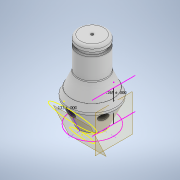
# Autodesk Inventor part: piston badflowchannel-1-16in-thread - neutron - 65flowchan
Saved by Autodesk Inventor 2020 (Build 240168000, 168)
## iProperties
Created: 2022-01-16
Part Number: piston badflowchannel-1-16in-thread - neutron - 65flowchan
Material: Generic
Document SubType Name: Modeling
Designer: pab2
Density: 1 g/cm^3
Appearance: Default
Author: pab2
Autodesk Inventor part; units mm, degrees
ref_plane "YZ Plane" through (0, 0, 0) normal (1, 0, 0) x (0, 1, 0)
ref_plane "XZ Plane" through (0, 0, 0) normal (0, 1, 0) x (-1, 0, 0)
ref_plane "XY Plane" through (0, 0, 0) normal (0, 0, 1) x (1, 0, 0)
sketch "Sketch1" plane through (0, 0, 0) normal (0, 0, 1) x (1, 0, 0)
  line L0 (0, 0) -> (8.4519, 0)
  line L1 (8.4519, 0) -> (8.4519, 12.7)
  line L2 (8.4519, 12.7) -> (7.0041, 12.7)
  line L3 (7.0041, 12.7) -> (7.0041, 15.113)
  line L4 (7.0041, 15.113) -> (8.4519, 15.113)
  line L5 (8.4519, 15.113) -> (8.4519, 18.288)
  line L6 (8.4519, 18.288) -> (0, 18.288)
  line L7 (0, 18.288) -> (0, 0)
  line L8 (0, -36.8534) -> (0, 27.4782) projected
  line L9 (8.4519, 0) -> (8.4519, 6.35)
  line L10 (8.4519, 0) -> (8.4519, 6.35)
  line L11 (8.4519, 6.35) -> (15.4293, -8.6131)
  line L12 (8.4519, 6.35) -> (24.9619, 6.35) construction
  line L13 (15.4293, -8.6131) -> (12.2543, -8.6131)
  line L14 (12.2543, -8.6131) -> (8.4519, 0)
  line L15 (15.4293, -8.6131) -> (0, -8.6131)
  line L16 (0, 0) -> (8.4519, 0)
  line L17 (0, -8.6131) -> (19.05, -8.6131)
  line L18 (19.05, -8.6131) -> (19.05, -27.6631)
  line L19 (19.05, -27.6631) -> (0, -27.6631)
  line L20 (0, -27.6631) -> (0, -8.6131)
  line L21 (19.05, -8.6131) -> (19.05, -16.3778)
  line L22 (7.3425, -27.6631) -> (12.7256, -16.1191)
  line L23 (7.3425, -27.6631) -> (20.0799, -27.6631) construction
  line L24 (8.4519, 0) -> (19.05, -23.5323)
  line L25 (14.2444, -12.862) -> (7.3425, -27.6631)
  point P0 (12.2543, -8.6131)
  point P1 (12.3309, -8.6131)
  dimension "d0" = 8.4519
  dimension "d1" = 12.7
  dimension "d2" = 90
  dimension "d3" = 1.4478
  dimension "d4" = 2.413
  dimension "d5" = 3.175
  dimension "d23" = 16.51
  dimension "d24" = 65
  dimension "d25" = 3.175
  dimension "d83" = 19.05
  dimension "d84" = 19.05
  dimension "d253" = 65
  constraints: 50 end point, 8 perpendicular, 8 point on line, 4 horizontal, 3 parallel, 2 collinear, 2 equal length, 2 vertical, 1 midpoint
  measures "d0" distance of L0.start L0.end
  measures "d1" distance of L0.end L1.end
  measures "d2" angle of L1 L0
  measures "d3" distance of L1.end L2.end
  measures "d4" distance of L2.end L3.end
  measures "d5" distance of L4.end L5.end
  measures "d23" distance of L9.end L11.end
  measures "d24" angle of L11 L12
  measures "d25" distance of L11.end L13.end
  measures "d83" distance of L18.end L19.end
  measures "d84" distance of L17.end L18.end
  measures "d253" angle of L23 L22
revolve "Revolution1" add sketch "Sketch1" angle 360 about axis through (0, -10, 0) along (0, 1, 0) contours L7 L6 L5 L4 L3 L2 L1 L0 | L0 L14 L15 L8 | L15 L13 L24 L25 L22 L19 L8
sketch "Sketch12" plane through (0, 18.288, 0) normal (0, 1, 0) x (1, 0, 0)
  point P0 (0, 0)
  point P1 (0, 0)
  constraints: 1 coincident
hole "Hole4" at (0, 18.288, 0) direction (0, -1, 0) diameter 1.5875 depth 27.94 tip angle 118
sketch "Sketch16" plane through (0, -27.6631, 0) normal (0, -1, 0) x (1, 0, 0)
  point P0 (0, 0)
hole "Hole8" at (0, -27.6631, 0) direction (0, 1, 0) diameter 4.9784 depth 6.35 thread size "1/4-20 UNC" class "2B" standard "ANSI Unified Screw Threads"
sketch "Sketch13" plane through (0, -27.6631, 0) normal (0, -1, 0) x (1, 0, 0)
  circle A0 centre (0, 0) radius 12.7 projected
  point P0 (12.7, 0)
  point P1 (0, -12.7)
  point P2 (-12.7, 0)
  point P3 (0, 12.7)
  constraints: 4 point on circle
ref_plane "Work Plane6" through (12.7, -21.3131, 0) normal (1, 0, 0) x (0, 1, 0)
sketch "Sketch14" plane through (12.7, -21.3131, 0) normal (1, 0, 0) x (0, 1, 0)
  line L0 (0, 12.7) -> (0, -12.7) projected
  line L1 (0, 0) -> (18.553, 0)
  line L2 (18.553, 12.7) -> (18.553, -12.7) projected
  line L3 (18.553, 0) -> (11.8347, 0)
  point P0 (21.3131, 0)
  dimension "d92" = 6.7183
  constraints: 4 end point, 2 midpoint, 1 point on line
  measures "d92" distance of L1.end L3.end
sketch "Sketch29" plane through (0, -27.6631, 0) normal (0, -1, 0) x (1, 0, 0)
  circle A0 centre (0, 0) radius 7.3425 projected
  point P0 (7.3425, 0)
  point P1 (0, -7.3425)
  point P2 (0, 7.3425)
  point P3 (-7.3425, 0)
  constraints: 4 point on circle
ref_plane "Work Plane5" through (0, -27.6631, 7.3425) normal (0, -0.4226183, 0.9063078) x (1, 0, 0)
sketch "Sketch30" plane through (0, -27.6631, 7.3425) normal (0, -0.4226183, 0.9063078) x (1, 0, 0)
  ellipse E0 centre (0, 10.3113) end of major axis (14.2444, 10.3113) minor radius 6.02 projected
  ellipse E1 centre (0, -3.1031) end of major axis (7.3425, -3.1031) minor radius 3.1031 projected
  line L0 (0, 0) -> (0, 16.3313)
  line L1 (0, 16.3313) -> (0, 12.9658)
  point P0 (0, 21.9682)
  dimension "d254" = 3.3655
  constraints: 4 end point, 2 vertical alignment, 1 point on line, 1 vertical, 2 other
  measures "d254" distance of L0.end L1.end
hole "Hole9" at (0, -15.9121, 12.8221) direction (0, 0.4226183, -0.9063078) diameter 1.5875 depth 13.97
hole "Hole10" at (0, -15.9121, 12.8221) direction (0, 0.4226183, -0.9063078) diameter 5.3594 depth 6.35 thread size "1/4-28 UNF" class "2B" standard "ANSI Unified Screw Threads"
pattern_circular "Circular Pattern7" count 4 over 200 about axis through (0, -10, 0) along (0, 1, 0) of "Hole9", "Hole10"
fillet "Fillet1" radius 1.5875 1 edges at (-8.4519, 18.288, 0)
fillet "Fillet2" radius 1.5875 3 edges at (-7.3425, -27.6631, 0) (-8.4519, 0, 0) (-14.2444, -12.862, 0)
equation "\"d54\" = 55deg"
equation "\"Sketch7_Pitch\" = 0.90714"
equation "\"d72\" = 55deg"
equation "\"Sketch9_Pitch\" = 1.27"
equation "\"d137\" = 55deg"
equation "\"Sketch17_Pitch\" = 1.27"
equation "\"d155\" = 55deg"
equation "\"Sketch19_Pitch\" = 0.90714"
equation "\"d173\" = 55deg"
equation "\"Sketch21_Pitch\" = 0.90714"
equation "\"d191\" = 55deg"
equation "\"Sketch23_Pitch\" = 1.27"
equation "\"d221\" = 55deg"
equation "\"Sketch25_Pitch\" = 0.90714"
equation "\"d239\" = 55deg"
equation "\"Sketch27_Pitch\" = 1.27"
body "Solid1"
